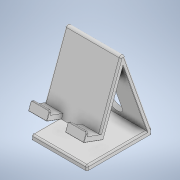
# Autodesk Inventor part: phone holder
Saved by Autodesk Inventor 2021 (Build 250183000, 183)
## iProperties
Created: 2020-09-28
Part Number: phone holder
Material: Generic
Document SubType Name: Modeling
Designer: cmzgt
Density: 1 g/cm^3
Appearance: Default
Author: cmzgt
## iProperties of the stored document _3DPrint.ipt
Created: 2020-09-28
Part Number: _3DPrint
Material: Generic
Document SubType Name: Modeling
Designer: cmzgt
Density: 1 g/cm^3
Appearance: Default
Author: cmzgt
Autodesk Inventor part; units mm, degrees
ref_plane "YZ Plane" through (0, 0, 0) normal (1, 0, 0) x (0, 1, 0)
ref_plane "XZ Plane" through (0, 0, 0) normal (0, 1, 0) x (-1, 0, 0)
ref_plane "XY Plane" through (0, 0, 0) normal (0, 0, 1) x (1, 0, 0)
sketch "Sketch1" plane through (0, 0, 0) normal (0, 1, 0) x (-1, 0, 0)
  line L0 (-38.1, -44.45) -> (38.1, -44.45)
  line L1 (38.1, -44.45) -> (38.1, 44.45)
  line L2 (38.1, 44.45) -> (-38.1, 44.45)
  line L3 (-38.1, 44.45) -> (-38.1, -44.45)
  line L4 (-38.1, -44.45) -> (38.1, 44.45) construction
  line L5 (38.1, -44.45) -> (-38.1, 44.45) construction
  point P0 (0, 0)
  dimension "d0" = 76.2
  dimension "d1" = 88.9
  constraints: 12 end point, 2 midpoint, 2 parallel, 1 horizontal, 1 perpendicular
  measures "d0" distance of L2.end L1.end
  measures "d1" distance of L1.end L0.end
extrude "Extrusion1" add sketch "Sketch1" along normal blind 6.35
sketch "Sketch2" plane through (38.1, 0, 44.45) normal (1, 0, 0) x (0, 0, -1)
  line L0 (88.9, 6.35) -> (0, 6.35) projected
  line L1 (88.9, 6.35) -> (49.3097, 118.9741)
  line L2 (88.9, 6.35) -> (82.55, 6.35)
  line L3 (49.3097, 118.9741) -> (15.9076, 28.418)
  line L4 (15.9076, 28.418) -> (21.8653, 26.2205)
  line L5 (21.8653, 26.2205) -> (49.361, 100.764)
  line L6 (49.361, 100.764) -> (82.55, 6.35)
  point P0 (44.45, 0)
  dimension "d12" = 119.38
  dimension "d13" = 6.35
  dimension "d14" = 96.52
  dimension "d15" = 6.35
  constraints: 12 end point, 2 parallel, 1 point on line
  measures "d12" distance of L0.start L1.end
  measures "d13" distance of L0.start L2.end
  measures "d14" distance of L1.end L3.end
  measures "d15" distance of L3.end L4.end
extrude "Extrusion2" add sketch "Sketch2" against normal blind 76.2
fillet "Fillet1" radius 3.175 1 edges at (0, 118.9741, -4.8597)
sketch "Sketch3" plane through (-38.1, 28.418, 28.5424) normal (0, 0.3460637, 0.938211) x (1, 0, 0)
  line L0 (76.2, 0) -> (76.2, 79.4529) projected
  line L1 (0, 0) -> (76.2, 0)
  line L2 (76.2, 0) -> (76.2, 6.35)
  line L3 (76.2, 6.35) -> (0, 6.35)
  line L4 (0, 6.35) -> (0, 0)
  point P0 (38.1, -16.7846)
  dimension "d19" = 6.35
  constraints: 8 end point, 2 parallel, 1 horizontal, 1 perpendicular, 1 point on line
  measures "d19" distance between parallel lines of L1 L3
extrude "Extrusion3" add sketch "Sketch3" along normal blind 21.59
sketch "Sketch4" plane through (-38.1, 34.3756, 26.3449) normal (0, 0.938211, -0.3460637) x (1, 0, 0)
  line L0 (76.2, -21.59) -> (0, -21.59) projected
  line L1 (76.2, -21.59) -> (76.2, 6.35) projected
  line L2 (0, -21.59) -> (76.2, -21.59)
  line L3 (76.2, -21.59) -> (76.2, -19.05)
  line L4 (76.2, -19.05) -> (0, -19.05)
  line L5 (0, -19.05) -> (0, -21.59)
  point P0 (38.1, 36.6132)
  dimension "d22" = 2.54
  constraints: 8 end point, 2 parallel, 1 horizontal, 1 perpendicular, 1 point on line
  measures "d22" distance of L3.end L2.end
extrude "Extrusion4" add sketch "Sketch4" along normal blind 5.08
sketch "Sketch5" plane through (-38.1, 35.8895, 48.7983) normal (0, 0.3460637, 0.938211) x (1, 0, 0)
  line L0 (0, 0) -> (76.2, 0) projected
  line L1 (0, 11.43) -> (76.2, 11.43) projected
  line L2 (25.3957, 0) -> (50.7957, 0)
  line L3 (50.7957, 0) -> (50.7957, 11.43)
  line L4 (50.7957, 11.43) -> (25.3957, 11.43)
  line L5 (25.3957, 11.43) -> (25.3957, 0)
  line L6 (0, 0) -> (0, 11.43) projected
  line L7 (76.2, 0) -> (76.2, 11.43) projected
  point P0 (38.1, -16.7846)
  point P1 (25.3957, 11.43)
  point P2 (50.7957, 0)
  dimension "d25" = 25.4
  dimension "d27" = 25.4043
  dimension "d28" = 25.3957
  constraints: 8 end point, 4 parallel, 2 point on line, 1 horizontal, 1 perpendicular
  measures "d25" distance of L3.end L4.end
  measures "d27" distance between parallel lines of L3 L7
  measures "d28" distance between parallel lines of L6 L5
extrude "Extrusion5" cut sketch "Sketch5" against normal up to surface (21.59 mm away) contours L5 L1 L3 L0
fillet "Fillet2" radius 2.032 7 edges at (38.1, 6.35, 3.175) (0, 6.35, 44.45) (-38.1, 6.35, 3.175) (38.1, 3.175, -44.45) (38.1, 3.175, 44.45) (-38.1, 3.175, 44.45) (-38.1, 3.175, -44.45)
fillet "Fillet3" radius 2.032 4 edges at (38.1, 46.1738, 43.6513) (12.6957, 46.1738, 43.6513) (-12.7043, 46.1738, 43.6513) (-38.1, 46.1738, 43.6513)
fillet "Fillet4" radius 0.508 10 edges at (-13.2995, 46.0549, 45.0488) (-12.7043, 40.2982, 47.1722) (-37.5048, 46.0549, 45.0488) (-38.1, 40.2982, 47.1722) (-25.4022, 46.6133, 44.8428) (37.5048, 46.0549, 45.0488) (38.1, 40.2982, 47.1722) (13.2908, 46.0549, 45.0488) (12.6957, 40.2982, 47.1722) (25.3978, 46.6133, 44.8428)
fillet "Fillet5" radius 2.032 9 edges at (-37.5048, 8.0431, -43.8548) (-38.1, 61.3941, -25.1006) (-38.1, 112.7796, -4.8122) (-38.1, 72.5395, 12.2679) (37.5048, 8.0431, -43.8548) (38.1, 61.3941, -25.1006) (38.1, 112.7796, -4.8122) (38.1, 72.5395, 12.2679) (0, 6.35, -44.45)
sketch "Sketch6" plane through (36.068, 110.6576, -7.7832) normal (0, 0.3316327, -0.9434086) x (-1, 0, 0)
  line L0 (36.068, -101.8142) -> (36.068, -51.0142) construction
  line L1 (45.593, -92.2892) -> (45.593, -60.5392)
  line L2 (26.543, -60.5392) -> (26.543, -92.2892)
  arc A0 (26.543, -92.2892) -> (45.593, -92.2892) centre (36.068, -92.2892) ccw
  arc A1 (45.593, -60.5392) -> (26.543, -60.5392) centre (36.068, -60.5392) ccw
  point P0 (36.068, -76.4142)
  dimension "d35" = 50.8
  dimension "d36" = 19.05
  constraints: 8 end point, 6 point on circle, 4 tangent, 2 centre point, 2 point on line, 1 midpoint, 1 parallel, 1 vertical
  measures "d35" distance of L0.start L0.end
  measures "d36" diameter of A1
extrude "Extrusion6" cut sketch "Sketch6" against normal up to next
fillet "Fillet6" radius 0.508 5 edges at (37.9512, 35.838, 48.6588) (38.1, 30.9671, 35.4532) (12.8445, 35.838, 48.6588) (12.6957, 32.0658, 38.4321) (25.3978, 35.8895, 48.7983)
fillet "Fillet7" radius 0.508 5 edges at (-12.8531, 35.838, 48.6588) (-12.7043, 32.0658, 38.4321) (-37.9512, 35.838, 48.6588) (-38.1, 30.9671, 35.4532) (-25.4022, 35.8895, 48.7983)
fillet "Fillet8" radius 0.508 1 edges at (-38.1, 52.541, -21.8627)
fillet "Fillet9" radius 0.508 1 edges at (38.1, 52.541, -21.8627)
body "Solid1"
